Autodesk Fusion 360 part; units mm, degrees
note: some values were not read from the file. Chosen so that the rebuilt part matches the saved one: which bodies a step acts on. Set by a fixed rule: which sketch regions a step uses.
(part 6 of 6)
  spline S14 degree 5 poles (28.4182, 7.3721) (28.401, 7.3374) (28.3665, 7.2685) (28.3146, 7.1668) (28.2449, 7.0342) (28.157, 6.8738) (28.0682, 6.7185) (27.9785, 6.5686) (27.8878, 6.4239) (27.796, 6.2845) (27.7028, 6.1503) (27.6083, 6.0213) (27.5124, 5.8974) (27.4154, 5.7789) (27.3181, 5.6659) (27.2215, 5.559) (27.1271, 5.4587) (27.0359, 5.3653) (26.9485, 5.2792) (26.8646, 5.2) (26.7825, 5.127) (26.7002, 5.0594) (26.6169, 4.9965) (26.5338, 4.9388) (26.4561, 4.8881) (26.3912, 4.8473) (26.3448, 4.8184) (26.3177, 4.8012) (26.3011, 4.7914) (26.2792, 4.7817) (26.2337, 4.7638) (26.1495, 4.7307) (26.0155, 4.6776) (25.8242, 4.6008) (25.5709, 4.4983) (25.2528, 4.3688) (24.9457, 4.2431) (24.6857, 4.1365) (24.4991, 4.0599) (24.4026, 4.0202) knots 0 0 0 0 0 0 0.028571 0.057143 0.085714 0.114286 0.142857 0.171429 0.2 0.228571 0.257143 0.285714 0.314286 0.342857 0.371429 0.4 0.428571 0.457143 0.485714 0.514286 0.542857 0.571429 0.6 0.628571 0.657143 0.685714 0.714286 0.742857 0.771429 0.8 0.828571 0.857143 0.885714 0.914286 0.942857 0.971429 1 1 1 1 1 1
  arc A14 (24.4026, 4.0202) -> (27.8435, 8.3674) centre (25.5471, 6.6497) ccw
  spline S15 degree 5 poles (27.8435, 8.3674) (27.8048, 8.3699) (27.728, 8.3745) (27.6139, 8.3804) (27.4643, 8.3863) (27.2813, 8.3904) (27.1025, 8.3911) (26.9278, 8.3884) (26.7572, 8.3822) (26.5906, 8.3724) (26.4277, 8.3588) (26.2687, 8.3415) (26.1135, 8.3203) (25.9623, 8.2956) (25.8159, 8.2678) (25.675, 8.2376) (25.5409, 8.206) (25.4145, 8.1737) (25.2962, 8.1411) (25.1857, 8.108) (25.0814, 8.0734) (24.9816, 8.036) (24.8855, 7.9953) (24.794, 7.9522) (24.7113, 7.9102) (24.6435, 7.8744) (24.5952, 7.8487) (24.5668, 7.8338) (24.55, 7.8243) (24.5306, 7.8102) (24.4924, 7.7798) (24.4217, 7.7234) (24.3086, 7.6339) (24.1465, 7.5067) (23.9311, 7.3385) (23.6599, 7.1278) (23.3975, 6.9247) (23.1752, 6.7528) (23.0155, 6.6295) (22.9329, 6.5658) knots 0 0 0 0 0 0 0.028571 0.057143 0.085714 0.114286 0.142857 0.171429 0.2 0.228571 0.257143 0.285714 0.314286 0.342857 0.371429 0.4 0.428571 0.457143 0.485714 0.514286 0.542857 0.571429 0.6 0.628571 0.657143 0.685714 0.714286 0.742857 0.771429 0.8 0.828571 0.857143 0.885714 0.914286 0.942857 0.971429 1 1 1 1 1 1
  arc A15 (22.8674, 13.3435) -> (22.9329, 6.5658) centre (25.8024, 9.9826) ccw
  spline S16 degree 5 poles (22.8674, 13.3435) (22.8699, 13.3048) (22.8745, 13.228) (22.8804, 13.1139) (22.8863, 12.9643) (22.8904, 12.7813) (22.8911, 12.6025) (22.8884, 12.4278) (22.8822, 12.2572) (22.8724, 12.0906) (22.8588, 11.9277) (22.8415, 11.7687) (22.8203, 11.6135) (22.7956, 11.4623) (22.7678, 11.3159) (22.7376, 11.175) (22.706, 11.0409) (22.6737, 10.9145) (22.6411, 10.7962) (22.608, 10.6857) (22.5734, 10.5814) (22.536, 10.4816) (22.4953, 10.3855) (22.4522, 10.294) (22.4102, 10.2113) (22.3744, 10.1435) (22.3487, 10.0952) (22.3338, 10.0668) (22.3243, 10.05) (22.3102, 10.0306) (22.2798, 9.9924) (22.2234, 9.9217) (22.1339, 9.8086) (22.0067, 9.6465) (21.8385, 9.4311) (21.6278, 9.1599) (21.4247, 8.8975) (21.2528, 8.6752) (21.1295, 8.5155) (21.0658, 8.4329) knots 0 0 0 0 0 0 0.028571 0.057143 0.085714 0.114286 0.142857 0.171429 0.2 0.228571 0.257143 0.285714 0.314286 0.342857 0.371429 0.4 0.428571 0.457143 0.485714 0.514286 0.542857 0.571429 0.6 0.628571 0.657143 0.685714 0.714286 0.742857 0.771429 0.8 0.828571 0.857143 0.885714 0.914286 0.942857 0.971429 1 1 1 1 1 1
  arc A16 (21.0658, 8.4329) -> (21.8721, 13.9182) centre (20.7422, 11.2823) ccw
  spline S17 degree 5 poles (21.8721, 13.9182) (21.8374, 13.901) (21.7685, 13.8665) (21.6668, 13.8146) (21.5342, 13.7449) (21.3738, 13.657) (21.2185, 13.5682) (21.0686, 13.4785) (20.9239, 13.3878) (20.7845, 13.296) (20.6503, 13.2028) (20.5213, 13.1083) (20.3974, 13.0124) (20.2789, 12.9154) (20.1659, 12.8181) (20.059, 12.7215) (19.9587, 12.6271) (19.8653, 12.5359) (19.7792, 12.4485) (19.7, 12.3646) (19.627, 12.2825) (19.5594, 12.2002) (19.4965, 12.1169) (19.4388, 12.0338) (19.3881, 11.9561) (19.3473, 11.8912) (19.3184, 11.8448) (19.3012, 11.8177) (19.2914, 11.8011) (19.2817, 11.7792) (19.2638, 11.7337) (19.2307, 11.6495) (19.1776, 11.5155) (19.1008, 11.3242) (18.9983, 11.0709) (18.8688, 10.7528) (18.7431, 10.4457) (18.6365, 10.1857) (18.5599, 9.9991) (18.5202, 9.9026) knots 0 0 0 0 0 0 0.028571 0.057143 0.085714 0.114286 0.142857 0.171429 0.2 0.228571 0.257143 0.285714 0.314286 0.342857 0.371429 0.4 0.428571 0.457143 0.485714 0.514286 0.542857 0.571429 0.6 0.628571 0.657143 0.685714 0.714286 0.742857 0.771429 0.8 0.828571 0.857143 0.885714 0.914286 0.942857 0.971429 1 1 1 1 1 1
  arc A17 (15.0747, 15.7395) -> (18.5202, 9.9026) centre (19.2968, 14.2964) ccw
  spline S18 degree 5 poles (15.0747, 15.7395) (15.0961, 15.7073) (15.1386, 15.643) (15.2007, 15.5472) (15.2807, 15.4206) (15.3756, 15.2642) (15.4657, 15.1097) (15.5507, 14.957) (15.6306, 14.8062) (15.7054, 14.6569) (15.7751, 14.5092) (15.8396, 14.3627) (15.8989, 14.2177) (15.953, 14.0745) (16.0022, 13.9337) (16.0465, 13.7967) (16.0862, 13.6647) (16.1214, 13.5391) (16.1523, 13.4203) (16.1789, 13.3081) (16.2011, 13.2004) (16.2185, 13.0953) (16.2313, 12.9918) (16.2398, 12.891) (16.2448, 12.7983) (16.2477, 12.7217) (16.2495, 12.6671) (16.2509, 12.635) (16.2511, 12.6158) (16.2485, 12.5919) (16.2413, 12.5436) (16.2278, 12.4541) (16.2069, 12.3115) (16.1777, 12.1075) (16.1398, 11.8368) (16.0929, 11.4966) (16.0482, 11.1678) (16.0105, 10.8893) (15.9836, 10.6894) (15.9697, 10.586) knots 0 0 0 0 0 0 0.028571 0.057143 0.085714 0.114286 0.142857 0.171429 0.2 0.228571 0.257143 0.285714 0.314286 0.342857 0.371429 0.4 0.428571 0.457143 0.485714 0.514286 0.542857 0.571429 0.6 0.628571 0.657143 0.685714 0.714286 0.742857 0.771429 0.8 0.828571 0.857143 0.885714 0.914286 0.942857 0.971429 1 1 1 1 1 1
  arc A18 (15.9697, 10.586) -> (13.9253, 15.7395) centre (14.2647, 12.8919) ccw
  spline S19 degree 5 poles (13.9253, 15.7395) (13.9039, 15.7073) (13.8614, 15.643) (13.7993, 15.5472) (13.7193, 15.4206) (13.6244, 15.2642) (13.5343, 15.1097) (13.4493, 14.957) (13.3694, 14.8062) (13.2946, 14.6569) (13.2249, 14.5092) (13.1604, 14.3627) (13.1011, 14.2177) (13.047, 14.0745) (12.9978, 13.9337) (12.9535, 13.7967) (12.9138, 13.6647) (12.8786, 13.5391) (12.8477, 13.4203) (12.8211, 13.3081) (12.7989, 13.2004) (12.7815, 13.0953) (12.7687, 12.9918) (12.7602, 12.891) (12.7552, 12.7983) (12.7523, 12.7217) (12.7505, 12.6671) (12.7491, 12.635) (12.7489, 12.6158) (12.7515, 12.5919) (12.7587, 12.5436) (12.7722, 12.4541) (12.7931, 12.3115) (12.8223, 12.1075) (12.8602, 11.8368) (12.9071, 11.4966) (12.9518, 11.1678) (12.9895, 10.8893) (13.0164, 10.6894) (13.0303, 10.586) knots 0 0 0 0 0 0 0.028571 0.057143 0.085714 0.114286 0.142857 0.171429 0.2 0.228571 0.257143 0.285714 0.314286 0.342857 0.371429 0.4 0.428571 0.457143 0.485714 0.514286 0.542857 0.571429 0.6 0.628571 0.657143 0.685714 0.714286 0.742857 0.771429 0.8 0.828571 0.857143 0.885714 0.914286 0.942857 0.971429 1 1 1 1 1 1
  arc A19 (7.1279, 13.9182) -> (13.0303, 10.586) centre (11.506, 14.7795) ccw
  spline S20 degree 5 poles (7.1279, 13.9182) (7.1626, 13.901) (7.2315, 13.8665) (7.3332, 13.8146) (7.4658, 13.7449) (7.6262, 13.657) (7.7815, 13.5682) (7.9314, 13.4785) (8.0761, 13.3878) (8.2155, 13.296) (8.3497, 13.2028) (8.4787, 13.1083) (8.6026, 13.0124) (8.7211, 12.9154) (8.8341, 12.8181) (8.941, 12.7215) (9.0413, 12.6271) (9.1347, 12.5359) (9.2208, 12.4485) (9.3, 12.3646) (9.373, 12.2825) (9.4406, 12.2002) (9.5035, 12.1169) (9.5612, 12.0338) (9.6119, 11.9561) (9.6527, 11.8912) (9.6816, 11.8448) (9.6988, 11.8177) (9.7086, 11.8011) (9.7183, 11.7792) (9.7362, 11.7337) (9.7693, 11.6495) (9.8224, 11.5155) (9.8992, 11.3242) (10.0017, 11.0709) (10.1312, 10.7528) (10.2569, 10.4457) (10.3635, 10.1857) (10.4401, 9.9991) (10.4798, 9.9026) knots 0 0 0 0 0 0 0.028571 0.057143 0.085714 0.114286 0.142857 0.171429 0.2 0.228571 0.257143 0.285714 0.314286 0.342857 0.371429 0.4 0.428571 0.457143 0.485714 0.514286 0.542857 0.571429 0.6 0.628571 0.657143 0.685714 0.714286 0.742857 0.771429 0.8 0.828571 0.857143 0.885714 0.914286 0.942857 0.971429 1 1 1 1 1 1
  arc A20 (10.4798, 9.9026) -> (6.1326, 13.3435) centre (7.8503, 11.0471) ccw
  spline S21 degree 5 poles (6.1326, 13.3435) (6.1301, 13.3048) (6.1255, 13.228) (6.1196, 13.1139) (6.1137, 12.9643) (6.1096, 12.7813) (6.1089, 12.6025) (6.1116, 12.4278) (6.1178, 12.2572) (6.1276, 12.0906) (6.1412, 11.9277) (6.1585, 11.7687) (6.1797, 11.6135) (6.2044, 11.4623) (6.2322, 11.3159) (6.2624, 11.175) (6.294, 11.0409) (6.3263, 10.9145) (6.3589, 10.7962) (6.392, 10.6857) (6.4266, 10.5814) (6.464, 10.4816) (6.5047, 10.3855) (6.5478, 10.294) (6.5898, 10.2113) (6.6256, 10.1435) (6.6513, 10.0952) (6.6662, 10.0668) (6.6757, 10.05) (6.6898, 10.0306) (6.7202, 9.9924) (6.7766, 9.9217) (6.8661, 9.8086) (6.9933, 9.6465) (7.1615, 9.4311) (7.3722, 9.1599) (7.5753, 8.8975) (7.7472, 8.6752) (7.8705, 8.5155) (7.9342, 8.4329) knots 0 0 0 0 0 0 0.028571 0.057143 0.085714 0.114286 0.142857 0.171429 0.2 0.228571 0.257143 0.285714 0.314286 0.342857 0.371429 0.4 0.428571 0.457143 0.485714 0.514286 0.542857 0.571429 0.6 0.628571 0.657143 0.685714 0.714286 0.742857 0.771429 0.8 0.828571 0.857143 0.885714 0.914286 0.942857 0.971429 1 1 1 1 1 1
  arc A21 (1.1565, 8.3674) -> (7.9342, 8.4329) centre (4.5174, 11.3024) ccw
  spline S22 degree 5 poles (1.1565, 8.3674) (1.1952, 8.3699) (1.272, 8.3745) (1.3861, 8.3804) (1.5357, 8.3863) (1.7187, 8.3904) (1.8975, 8.3911) (2.0722, 8.3884) (2.2428, 8.3822) (2.4094, 8.3724) (2.5723, 8.3588) (2.7313, 8.3415) (2.8865, 8.3203) (3.0377, 8.2956) (3.1841, 8.2678) (3.325, 8.2376) (3.4591, 8.206) (3.5855, 8.1737) (3.7038, 8.1411) (3.8143, 8.108) (3.9186, 8.0734) (4.0184, 8.036) (4.1145, 7.9953) (4.206, 7.9522) (4.2887, 7.9102) (4.3565, 7.8744) (4.4048, 7.8487) (4.4332, 7.8338) (4.45, 7.8243) (4.4694, 7.8102) (4.5076, 7.7798) (4.5783, 7.7234) (4.6914, 7.6339) (4.8535, 7.5067) (5.0689, 7.3385) (5.3401, 7.1278) (5.6025, 6.9247) (5.8248, 6.7528) (5.9845, 6.6295) (6.0671, 6.5658) knots 0 0 0 0 0 0 0.028571 0.057143 0.085714 0.114286 0.142857 0.171429 0.2 0.228571 0.257143 0.285714 0.314286 0.342857 0.371429 0.4 0.428571 0.457143 0.485714 0.514286 0.542857 0.571429 0.6 0.628571 0.657143 0.685714 0.714286 0.742857 0.771429 0.8 0.828571 0.857143 0.885714 0.914286 0.942857 0.971429 1 1 1 1 1 1
  arc A22 (6.0671, 6.5658) -> (0.5818, 7.3721) centre (3.2177, 6.2422) ccw
  spline S23 degree 5 poles (0.5818, 7.3721) (0.599, 7.3374) (0.6335, 7.2685) (0.6854, 7.1668) (0.7551, 7.0342) (0.843, 6.8738) (0.9318, 6.7185) (1.0215, 6.5686) (1.1122, 6.4239) (1.204, 6.2845) (1.2972, 6.1503) (1.3917, 6.0213) (1.4876, 5.8974) (1.5846, 5.7789) (1.6819, 5.6659) (1.7785, 5.559) (1.8729, 5.4587) (1.9641, 5.3653) (2.0515, 5.2792) (2.1354, 5.2) (2.2175, 5.127) (2.2998, 5.0594) (2.3831, 4.9965) (2.4662, 4.9388) (2.5439, 4.8881) (2.6088, 4.8473) (2.6552, 4.8184) (2.6823, 4.8012) (2.6989, 4.7914) (2.7208, 4.7817) (2.7663, 4.7638) (2.8505, 4.7307) (2.9845, 4.6776) (3.1758, 4.6008) (3.4291, 4.4983) (3.7472, 4.3688) (4.0543, 4.2431) (4.3143, 4.1365) (4.5009, 4.0599) (4.5974, 4.0202) knots 0 0 0 0 0 0 0.028571 0.057143 0.085714 0.114286 0.142857 0.171429 0.2 0.228571 0.257143 0.285714 0.314286 0.342857 0.371429 0.4 0.428571 0.457143 0.485714 0.514286 0.542857 0.571429 0.6 0.628571 0.657143 0.685714 0.714286 0.742857 0.771429 0.8 0.828571 0.857143 0.885714 0.914286 0.942857 0.971429 1 1 1 1 1 1
  arc A23 (-1.2395, 0.5747) -> (4.5974, 4.0202) centre (0.2036, 4.7968) ccw
  point P0 (-0.3392, 1.1124)
  point P1 (0.4456, 1.4593)
  point P2 (1.0843, 1.6528)
  point P3 (1.5538, 1.7347)
  point P4 (1.8395, 1.7498)
  point P5 (1.9347, 1.7445)
  point P6 (-0.3392, -1.1124)
  point P7 (0.4456, -1.4593)
  point P8 (1.0843, -1.6528)
  point P9 (1.5538, -1.7347)
  point P10 (1.8395, -1.7498)
  point P11 (1.9347, -1.7445)
  point P12 (1.0927, -6.4562)
  point P13 (1.5989, -5.7634)
  point P14 (2.0552, -5.2765)
  point P15 (2.4209, -4.9708)
  point P16 (2.6607, -4.8149)
  point P17 (2.7459, -4.7719)
  point P18 (2.2051, -8.383)
  point P19 (3.0582, -8.291)
  point P20 (3.708, -8.1392)
  point P21 (4.1557, -7.9754)
  point P22 (4.4106, -7.8457)
  point P23 (4.4903, -7.7934)
  point P24 (6.117, -12.2949)
  point P25 (6.209, -11.4418)
  point P26 (6.3608, -10.792)
  point P27 (6.5246, -10.3443)
  point P28 (6.6543, -10.0894)
  point P29 (6.7066, -10.0097)
  point P30 (8.0438, -13.4073)
  point P31 (8.7366, -12.9011)
  point P32 (9.2235, -12.4448)
  point P33 (9.5292, -12.0791)
  point P34 (9.6851, -11.8393)
  point P35 (9.7281, -11.7541)
  point P36 (13.3876, -14.8392)
  point P37 (13.0407, -14.0544)
  point P38 (12.8472, -13.4157)
  point P39 (12.7653, -12.9462)
  point P40 (12.7502, -12.6605)
  point P41 (12.7555, -12.5653)
  point P42 (15.6124, -14.8392)
  point P43 (15.9593, -14.0544)
  point P44 (16.1528, -13.4157)
  point P45 (16.2347, -12.9462)
  point P46 (16.2498, -12.6605)
  point P47 (16.2445, -12.5653)
  point P48 (20.9562, -13.4073)
  point P49 (20.2634, -12.9011)
  point P50 (19.7765, -12.4448)
  point P51 (19.4708, -12.0791)
  point P52 (19.3149, -11.8393)
  point P53 (19.2719, -11.7541)
  point P54 (22.883, -12.2949)
  point P55 (22.791, -11.4418)
  point P56 (22.6392, -10.792)
  point P57 (22.4754, -10.3443)
  point P58 (22.3457, -10.0894)
  point P59 (22.2934, -10.0097)
  point P60 (26.7949, -8.383)
  point P61 (25.9418, -8.291)
  point P62 (25.292, -8.1392)
  point P63 (24.8443, -7.9754)
  point P64 (24.5894, -7.8457)
  point P65 (24.5097, -7.7934)
  point P66 (27.9073, -6.4562)
  point P67 (27.4011, -5.7634)
  point P68 (26.9448, -5.2765)
  point P69 (26.5791, -4.9708)
  point P70 (26.3393, -4.8149)
  point P71 (26.2541, -4.7719)
  point P72 (29.3392, -1.1124)
  point P73 (28.5544, -1.4593)
  point P74 (27.9157, -1.6528)
  point P75 (27.4462, -1.7347)
  point P76 (27.1605, -1.7498)
  point P77 (27.0653, -1.7445)
  point P78 (29.3392, 1.1124)
  point P79 (28.5544, 1.4593)
  point P80 (27.9157, 1.6528)
  point P81 (27.4462, 1.7347)
  point P82 (27.1605, 1.7498)
  point P83 (27.0653, 1.7445)
  point P84 (27.9073, 6.4562)
  point P85 (27.4011, 5.7634)
  point P86 (26.9448, 5.2765)
  point P87 (26.5791, 4.9708)
  point P88 (26.3393, 4.8149)
  point P89 (26.2541, 4.7719)
  point P90 (26.7949, 8.383)
  point P91 (25.9418, 8.291)
  point P92 (25.292, 8.1392)
  point P93 (24.8443, 7.9754)
  point P94 (24.5894, 7.8457)
  point P95 (24.5097, 7.7934)
  point P96 (22.883, 12.2949)
  point P97 (22.791, 11.4418)
  point P98 (22.6392, 10.792)
  point P99 (22.4754, 10.3443)
  point P100 (22.3457, 10.0894)
  point P101 (22.2934, 10.0097)
  point P102 (20.9562, 13.4073)
  point P103 (20.2634, 12.9011)
  point P104 (19.7765, 12.4448)
  point P105 (19.4708, 12.0791)
  point P106 (19.3149, 11.8393)
  point P107 (19.2719, 11.7541)
  point P108 (15.6124, 14.8392)
  point P109 (15.9593, 14.0544)
  point P110 (16.1528, 13.4157)
  point P111 (16.2347, 12.9462)
  point P112 (16.2498, 12.6605)
  point P113 (16.2445, 12.5653)
  point P114 (13.3876, 14.8392)
  point P115 (13.0407, 14.0544)
  point P116 (12.8472, 13.4157)
  point P117 (12.7653, 12.9462)
  point P118 (12.7502, 12.6605)
  point P119 (12.7555, 12.5653)
  point P120 (8.0438, 13.4073)
  point P121 (8.7366, 12.9011)
  point P122 (9.2235, 12.4448)
  point P123 (9.5292, 12.0791)
  point P124 (9.6851, 11.8393)
  point P125 (9.7281, 11.7541)
  point P126 (6.117, 12.2949)
  point P127 (6.209, 11.4418)
  point P128 (6.3608, 10.792)
  point P129 (6.5246, 10.3443)
  point P130 (6.6543, 10.0894)
  point P131 (6.7066, 10.0097)
  point P132 (2.2051, 8.383)
  point P133 (3.0582, 8.291)
  point P134 (3.708, 8.1392)
  point P135 (4.1557, 7.9754)
  point P136 (4.4106, 7.8457)
  point P137 (4.4903, 7.7934)
  point P138 (1.0927, 6.4562)
  point P139 (1.5989, 5.7634)
  point P140 (2.0552, 5.2765)
  point P141 (2.4209, 4.9708)
  point P142 (2.6607, 4.8149)
  point P143 (2.7459, 4.7719)
extrude "押し出し1''''''''''''''''" add sketch "スケッチ1 (17)" along normal blind 16 from surface at 66 separate body contours S0 A0 S1 A1 S2 A2 S3 A3 S4 A4 S5 A5 S6 A6 S7 A7 S8 A8 S9 A9 S10 A10 S11 A11 S12 A12 S13 A13 S14 A14 S15 A15 S16 A16 S17 A17 S18 A18 S19 A19 S20 A20 S21 A21 S22 A22 S23 A23 makes body 25 in component "Intermediate_Pinion_12T"
sketch "スケッチ2 (16)" plane through (0, 0, 0) normal (0, 0, 1) x (1, 0, 0) in component "Intermediate_Pinion_12T"
  circle A0 centre (14.5, 0) radius 9
extrude "押し出し2'''''''''''''''" add sketch "スケッチ2 (16)" along normal blind 4 from surface at 82 bodies 25 in component "Intermediate_Pinion_12T"
sketch "スケッチ3 (15)" plane through (0, 0, 0) normal (0, 0, 1) x (1, 0, 0) in component "Intermediate_Pinion_12T"
  circle A0 centre (14.5, 0) radius 5
extrude "押し出し3'''''''''''''" cut sketch "スケッチ3 (15)" along normal blind 30 from surface at 62 bodies 25 in component "Intermediate_Pinion_12T"
sketch "スケッチ1 (18)" plane through (0, 0, 0) normal (0, 0, 1) x (1, 0, 0) in component "Stage2_Driver_Disc"
  circle A0 centre (14.5, 0) radius 62
extrude "押し出し1'''''''''''''''''" add sketch "スケッチ1 (18)" along normal blind 14 from surface at 86 separate body makes body 26 in component "Stage2_Driver_Disc"
sketch "スケッチ2 (17)" plane through (0, 0, 0) normal (0, 0, 1) x (1, 0, 0) in component "Stage2_Driver_Disc"
  circle A0 centre (14.5, 0) radius 16
extrude "押し出し2''''''''''''''''" add sketch "スケッチ2 (17)" along normal blind 34 from surface at 86 bodies 26 in component "Stage2_Driver_Disc"
sketch "スケッチ3 (16)" plane through (0, 0, 0) normal (0, 0, 1) x (1, 0, 0) in component "Stage2_Driver_Disc"
  circle A0 centre (14.5, 0) radius 30
  circle A1 centre (-61.5, 0) radius 59
extrude "押し出し3''''''''''''''" add sketch "スケッチ3 (16)" along normal blind 20 from surface at 100 contours A0 A1 picked at (10.4448, -9.1222) bodies 26 in component "Stage2_Driver_Disc"
sketch "スケッチ4 (10)" plane through (0, 0, 0) normal (0, 0, 1) x (1, 0, 0) in component "Stage2_Driver_Disc"
  circle A0 centre (56.5, 0) radius 12
  circle A1 centre (14.5, 42) radius 12
  circle A2 centre (14.5, -42) radius 12
extrude "押し出し4''''''''" cut sketch "スケッチ4 (10)" along normal blind 14 from surface at 86 bodies 26 in component "Stage2_Driver_Disc"
sketch "スケッチ5 (8)" plane through (0, 0, 0) normal (0, 0, 1) x (1, 0, 0) in component "Stage2_Driver_Disc"
  circle A0 centre (14.5, 0) radius 5
extrude "押し出し5''''''" cut sketch "スケッチ5 (8)" along normal blind 42 from surface at 82 bodies 26 in component "Stage2_Driver_Disc"
sketch "スケッチ1 (19)" plane through (0, 0, 0) normal (0, 0, 1) x (1, 0, 0) in component "Stage2_Drive_Pin"
  circle A0 centre (-39.2401, 0) radius 6
extrude "押し出し1''''''''''''''''''" add sketch "スケッチ1 (19)" along normal blind 26 from surface at 100 separate body makes body 27 in component "Stage2_Drive_Pin"
sketch "スケッチ2 (18)" plane through (0, 0, 0) normal (0, 0, 1) x (1, 0, 0) in component "Stage2_Drive_Pin"
  circle A0 centre (-39.2401, 0) radius 9.5
extrude "押し出し2'''''''''''''''''" add sketch "スケッチ2 (18)" along normal blind 6 from surface at 120 bodies 27 in component "Stage2_Drive_Pin"
sketch "スケッチ1 (20)" plane through (0, 0, 0) normal (0, 0, 1) x (1, 0, 0) in component "Stage2_Geneva_Wheel_4Slot"
  circle A0 centre (90.5, 0) radius 58
extrude "押し出し1'''''''''''''''''''" add sketch "スケッチ1 (20)" along normal blind 12 from surface at 104 separate body makes body 28 in component "Stage2_Geneva_Wheel_4Slot"
sketch "スケッチ2 (19)" plane through (0, 0, 0) normal (0, 0, 1) x (1, 0, 0) in component "Stage2_Geneva_Wheel_4Slot"
  circle A0 centre (90.5, 0) radius 14
extrude "押し出し2''''''''''''''''''" add sketch "スケッチ2 (19)" along normal blind 18 from surface at 100 bodies 28 in component "Stage2_Geneva_Wheel_4Slot"
sketch "スケッチ3 (17)" plane through (0, 0, 0) normal (0, 0, 1) x (1, 0, 0) in component "Stage2_Geneva_Wheel_4Slot"
  line L0 (79.3561, -20.3363) -> (48.4271, -51.2652)
  line L1 (48.4271, -51.2652) -> (39.2348, -42.0729)
  line L2 (39.2348, -42.0729) -> (70.1637, -11.1439)
  arc A0 (79.3561, -20.3363) -> (70.1637, -11.1439) centre (74.7599, -15.7401) ccw
  line L3 (110.8363, -11.1439) -> (141.7652, -42.0729)
  line L4 (141.7652, -42.0729) -> (132.5729, -51.2652)
  line L5 (132.5729, -51.2652) -> (101.6439, -20.3363)
  arc A1 (110.8363, -11.1439) -> (101.6439, -20.3363) centre (106.2401, -15.7401) ccw
  line L6 (101.6439, 20.3363) -> (132.5729, 51.2652)
  line L7 (132.5729, 51.2652) -> (141.7652, 42.0729)
  line L8 (141.7652, 42.0729) -> (110.8363, 11.1439)
  arc A2 (101.6439, 20.3363) -> (110.8363, 11.1439) centre (106.2401, 15.7401) ccw
  line L9 (70.1637, 11.1439) -> (39.2348, 42.0729)
  line L10 (39.2348, 42.0729) -> (48.4271, 51.2652)
  line L11 (48.4271, 51.2652) -> (79.3561, 20.3363)
  arc A3 (70.1637, 11.1439) -> (79.3561, 20.3363) centre (74.7599, 15.7401) ccw
extrude "押し出し3'''''''''''''''" cut sketch "スケッチ3 (17)" along normal blind 20 from surface at 100 bodies 28 in component "Stage2_Geneva_Wheel_4Slot"
sketch "スケッチ4 (11)" plane through (0, 0, 0) normal (0, 0, 1) x (1, 0, 0) in component "Stage2_Geneva_Wheel_4Slot"
  circle A0 centre (166.5, 0) radius 30
  circle A1 centre (90.5, 76) radius 30
  circle A2 centre (14.5, 0) radius 30
  circle A3 centre (90.5, -76) radius 30
extrude "押し出し4'''''''''" cut sketch "スケッチ4 (11)" along normal blind 20 from surface at 100 bodies 28 in component "Stage2_Geneva_Wheel_4Slot"
sketch "スケッチ5 (9)" plane through (0, 0, 0) normal (0, 0, 1) x (1, 0, 0) in component "Stage2_Geneva_Wheel_4Slot"
  circle A0 centre (123.5, 0) radius 9
  circle A1 centre (90.5, 33) radius 9
  circle A2 centre (57.5, 0) radius 9
  circle A3 centre (90.5, -33) radius 9
extrude "押し出し5'''''''" cut sketch "スケッチ5 (9)" along normal blind 20 from surface at 100 bodies 28 in component "Stage2_Geneva_Wheel_4Slot"
sketch "スケッチ6 (4)" plane through (0, 0, 0) normal (0, 0, 1) x (1, 0, 0) in component "Stage2_Geneva_Wheel_4Slot"
  circle A0 centre (90.5, 0) radius 8
extrude "押し出し6''" cut sketch "スケッチ6 (4)" along normal blind 26 from surface at 96 bodies 28 in component "Stage2_Geneva_Wheel_4Slot"
sketch "スケッチ1 (21)" plane through (0, 0, 0) normal (0, 0, 1) x (1, 0, 0) in component "Output_Index_Table"
  circle A0 centre (90.5, 0) radius 62
extrude "押し出し1''''''''''''''''''''" add sketch "スケッチ1 (21)" along normal blind 16 from surface at 132 separate body makes body 29 in component "Output_Index_Table"
sketch "スケッチ2 (20)" plane through (0, 0, 0) normal (0, 0, 1) x (1, 0, 0) in component "Output_Index_Table"
  circle A0 centre (90.5, 0) radius 22
extrude "押し出し2'''''''''''''''''''" add sketch "スケッチ2 (20)" along normal blind 14 from surface at 118 bodies 29 in component "Output_Index_Table"
sketch "スケッチ3 (18)" plane through (0, 0, 0) normal (0, 0, 1) x (1, 0, 0) in component "Output_Index_Table"
  circle A0 centre (142.5, 0) radius 7
  circle A1 centre (132.5689, 30.5648) radius 7
  circle A2 centre (106.5689, 49.4549) radius 7
  circle A3 centre (74.4311, 49.4549) radius 7
  circle A4 centre (48.4311, 30.5648) radius 7
  circle A5 centre (38.5, 0) radius 7
  circle A6 centre (48.4311, -30.5648) radius 7
  circle A7 centre (74.4311, -49.4549) radius 7
  circle A8 centre (106.5689, -49.4549) radius 7
  circle A9 centre (132.5689, -30.5648) radius 7
extrude "押し出し3''''''''''''''''" cut sketch "スケッチ3 (18)" along normal blind 24 from surface at 128 bodies 29 in component "Output_Index_Table"
sketch "スケッチ4 (12)" plane through (0, 0, 0) normal (0, 0, 1) x (1, 0, 0) in component "Output_Index_Table"
  circle A0 centre (90.5, 0) radius 43
  circle A1 centre (90.5, 0) radius 38
extrude "押し出し4''''''''''" cut sketch "スケッチ4 (12)" along normal blind 6 from surface at 143 bodies 29 in component "Output_Index_Table"
sketch "スケッチ5 (10)" plane through (0, 0, 0) normal (0, 0, 1) x (1, 0, 0) in component "Output_Index_Table"
  circle A0 centre (116.4808, 15) radius 3.5
  circle A1 centre (90.5, 30) radius 3.5
  circle A2 centre (64.5192, 15) radius 3.5
  circle A3 centre (64.5192, -15) radius 3.5
  circle A4 centre (90.5, -30) radius 3.5
  circle A5 centre (116.4808, -15) radius 3.5
extrude "押し出し5''''''''" cut sketch "スケッチ5 (10)" along normal blind 24 from surface at 128 bodies 29 in component "Output_Index_Table"
sketch "スケッチ6 (5)" plane through (0, 0, 0) normal (0, 0, 1) x (1, 0, 0) in component "Output_Index_Table"
  circle A0 centre (90.5, 0) radius 8
extrude "押し出し6'''" cut sketch "スケッチ6 (5)" along normal blind 40 from surface at 114 bodies 29 in component "Output_Index_Table"
sketch "スケッチ1 (22)" plane through (0, 0, 0) normal (0, 0, 1) x (1, 0, 0) in component "Upper_Support_Plate"
  line L0 (-290, -125) -> (200, -125)
  line L1 (200, -125) -> (200, 125)
  line L2 (200, 125) -> (-290, 125)
  line L3 (-290, 125) -> (-290, -125)
extrude "押し出し1'''''''''''''''''''''" add sketch "スケッチ1 (22)" along normal blind 12 from surface at 158 separate body makes body 30 in component "Upper_Support_Plate"
fillet "フィレット1'" radius 24 4 edges at (-290, 125, 164) (200, 125, 164) (200, -125, 164) (-290, -125, 164) on bodies 30 in component "Upper_Support_Plate"
sketch "スケッチ2 (21)" plane through (0, 0, 0) normal (0, 0, 1) x (1, 0, 0) in component "Upper_Support_Plate"
  circle A0 centre (-176, 0) radius 12
  circle A1 centre (-80, 0) radius 11
  circle A2 centre (14.5, 0) radius 8
  circle A3 centre (90.5, 0) radius 11
extrude "押し出し2''''''''''''''''''''" cut sketch "スケッチ2 (21)" along normal blind 20 from surface at 154 bodies 30 in component "Upper_Support_Plate"
sketch "スケッチ3 (19)" plane through (0, 0, 0) normal (0, 0, 1) x (1, 0, 0) in component "Upper_Support_Plate"
  circle A0 centre (-265, 105) radius 6.5
  circle A1 centre (-265, -105) radius 6.5
  circle A2 centre (-45, 107) radius 6.5
  circle A3 centre (-45, -107) radius 6.5
  circle A4 centre (100, 107) radius 6.5
  circle A5 centre (100, -107) radius 6.5
  circle A6 centre (175, 105) radius 6.5
  circle A7 centre (175, -105) radius 6.5
extrude "押し出し3'''''''''''''''''" cut sketch "スケッチ3 (19)" along normal blind 20 from surface at 154 bodies 30 in component "Upper_Support_Plate"
sketch "スケッチ4 (13)" plane through (0, 0, 0) normal (0, 0, 1) x (1, 0, 0) in component "Upper_Support_Plate"
  circle A0 centre (-230, 0) radius 26
  circle A1 centre (150, 0) radius 26
extrude "押し出し4'''''''''''" cut sketch "スケッチ4 (13)" along normal blind 20 from surface at 154 bodies 30 in component "Upper_Support_Plate"
sketch "スケッチ1 (23)" plane through (0, 0, 0) normal (0, 0, 1) x (1, 0, 0) in component "Upper_Bearing_Rings"
  circle A0 centre (-176, 0) radius 20
  circle A1 centre (-80, 0) radius 20
  circle A2 centre (14.5, 0) radius 20
  circle A3 centre (90.5, 0) radius 20
extrude "押し出し1''''''''''''''''''''''" add sketch "スケッチ1 (23)" along normal blind 14 from surface at 170 separate body makes body 31 at (34.4006, -1.9914, 179.3333) makes body 32 at (-60.0994, -1.9914, 179.3333) makes body 33 at (-156.0994, -1.9914, 179.3333) makes body 34 at (110.4006, -1.9914, 179.3333) in component "Upper_Bearing_Rings"
sketch "スケッチ2 (22)" plane through (0, 0, 0) normal (0, 0, 1) x (1, 0, 0) in component "Upper_Bearing_Rings"
  circle A0 centre (-176, 0) radius 25
  circle A1 centre (-80, 0) radius 25
  circle A2 centre (14.5, 0) radius 25
  circle A3 centre (90.5, 0) radius 25
extrude "押し出し2'''''''''''''''''''''" add sketch "スケッチ2 (22)" along normal blind 5 from surface at 170 bodies 31 32 33 34 in component "Upper_Bearing_Rings"
sketch "スケッチ3 (20)" plane through (0, 0, 0) normal (0, 0, 1) x (1, 0, 0) in component "Upper_Bearing_Rings"
  circle A0 centre (-176, 0) radius 10.5
  circle A1 centre (-80, 0) radius 9.5
  circle A2 centre (14.5, 0) radius 6.5
  circle A3 centre (90.5, 0) radius 9.5
extrude "押し出し3''''''''''''''''''" cut sketch "スケッチ3 (20)" along normal blind 22 from surface at 166 bodies 31 32 33 34 in component "Upper_Bearing_Rings"
sketch "スケッチ1 (24)" plane through (0, 0, 0) normal (0, 0, 1) x (1, 0, 0) in component "Standoff_Bolts"
  circle A0 centre (-265, 105) radius 5.8
  circle A1 centre (-265, -105) radius 5.8
  circle A2 centre (-45, 107) radius 5.8
  circle A3 centre (-45, -107) radius 5.8
  circle A4 centre (100, 107) radius 5.8
  circle A5 centre (100, -107) radius 5.8
  circle A6 centre (175, 105) radius 5.8
  circle A7 centre (175, -105) radius 5.8
extrude "押し出し1'''''''''''''''''''''''" add sketch "スケッチ1 (24)" along normal blind 24 from surface at 146 separate body makes body 35 at (178.3857, 109.7092, 162) makes body 36 at (105.7928, 106.7109, 162) makes body 37 at (-39.2072, -107.2891, 162) makes body 38 at (-260.3766, -101.4979, 162) makes body 39 at (-39.2072, 106.7109, 162) makes body 40 at (-260.3766, 108.5021, 162) makes body 41 at (105.7928, -107.2891, 162) makes body 42 at (178.3857, -100.2908, 162) in component "Standoff_Bolts"
sketch "スケッチ2 (23)" plane through (0, 0, 0) normal (0, 0, 1) x (1, 0, 0) in component "Standoff_Bolts"
  circle A0 centre (-265, 105) radius 14
  circle A1 centre (-265, -105) radius 14
  circle A2 centre (-45, 107) radius 14
  circle A3 centre (-45, -107) radius 14
  circle A4 centre (100, 107) radius 14
  circle A5 centre (100, -107) radius 14
  circle A6 centre (175, 105) radius 14
  circle A7 centre (175, -105) radius 14
extrude "押し出し2''''''''''''''''''''''" add sketch "スケッチ2 (23)" along normal blind 3 from surface at 170 bodies 35 36 37 38 39 40 41 42 in component "Standoff_Bolts"
sketch "スケッチ3 (21)" plane through (0, 0, 0) normal (0, 0, 1) x (1, 0, 0) in component "Standoff_Bolts"
  circle A0 centre (-265, 105) radius 10.5
  circle A1 centre (-265, -105) radius 10.5
  circle A2 centre (-45, 107) radius 10.5
  circle A3 centre (-45, -107) radius 10.5
  circle A4 centre (100, 107) radius 10.5
  circle A5 centre (100, -107) radius 10.5
  circle A6 centre (175, 105) radius 10.5
  circle A7 centre (175, -105) radius 10.5
extrude "押し出し3'''''''''''''''''''" add sketch "スケッチ3 (21)" along normal blind 8 from surface at 173 bodies 35 36 37 38 39 40 41 42 in component "Standoff_Bolts"
sketch "スケッチ1 (25)" plane through (0, 0, 0) normal (0, 0, 1) x (1, 0, 0) in component "Table_Fixing_Bolts"
  circle A0 centre (116.4808, 15) radius 3.4
  circle A1 centre (90.5, 30) radius 3.4
  circle A2 centre (64.5192, 15) radius 3.4
  circle A3 centre (64.5192, -15) radius 3.4
  circle A4 centre (90.5, -30) radius 3.4
  circle A5 centre (116.4808, -15) radius 3.4
extrude "押し出し1''''''''''''''''''''''''" add sketch "スケッチ1 (25)" along normal blind 18 from surface at 130 separate body makes body 43 at (93.8958, -30.1695, 142) makes body 44 at (119.8765, 14.8305, 142) makes body 45 at (93.8958, 29.8305, 142) makes body 46 at (67.915, 14.8305, 142) makes body 47 at (66.0704, -11.9744, 142) makes body 48 at (119.8765, -15.1695, 142) in component "Table_Fixing_Bolts"
sketch "スケッチ2 (24)" plane through (0, 0, 0) normal (0, 0, 1) x (1, 0, 0) in component "Table_Fixing_Bolts"
  circle A0 centre (116.4808, 15) radius 6
  circle A1 centre (90.5, 30) radius 6
  circle A2 centre (64.5192, 15) radius 6
  circle A3 centre (64.5192, -15) radius 6
  circle A4 centre (90.5, -30) radius 6
  circle A5 centre (116.4808, -15) radius 6
extrude "押し出し2'''''''''''''''''''''''" add sketch "スケッチ2 (24)" along normal blind 5 from surface at 148 bodies 43 44 45 46 47 48 in component "Table_Fixing_Bolts"
extrude "押し出し6''''" cut sketch "スケッチ3 (14)" along normal blind 5 from surface at 66 bodies 24 in component "Intermediate_Spur_Gear_72T"
component "Lower_Base_Plate" placed x (1, 0, 0) y (0, 1, 0) z (0, 0, 1) at (0, 0, 0)
component "Bearing_Housing_A" placed x (1, 0, 0) y (0, 1, 0) z (0, 0, 1) at (0, 0, 0)
component "Bearing_Housing_B" placed x (1, 0, 0) y (0, 1, 0) z (0, 0, 1) at (0, 0, 0)
component "Bearing_Housing_C" placed x (1, 0, 0) y (0, 1, 0) z (0, 0, 1) at (0, 0, 0)
component "Bearing_Housing_D" placed x (1, 0, 0) y (0, 1, 0) z (0, 0, 1) at (0, 0, 0)
component "Standoff_Posts" placed x (1, 0, 0) y (0, 1, 0) z (0, 0, 1) at (0, 0, 0)
component "Input_Shaft" placed x (1, 0, 0) y (0, 1, 0) z (0, 0, 1) at (0, 0, 0)
component "Stage1_Shaft" placed x (1, 0, 0) y (0, 1, 0) z (0, 0, 1) at (0, 0, 0)
component "Stage2_Driver_Shaft" placed x (1, 0, 0) y (0, 1, 0) z (0, 0, 1) at (0, 0, 0)
component "Output_Shaft" placed x (1, 0, 0) y (0, 1, 0) z (0, 0, 1) at (0, 0, 0)
component "Input_Handwheel" placed x (1, 0, 0) y (0, 1, 0) z (0, 0, 1) at (0, 0, 0)
component "Input_Crank_Handle" placed x (1, 0, 0) y (0, 1, 0) z (0, 0, 1) at (0, 0, 0)
component "Stage1_Driver_Disc" placed x (1, 0, 0) y (0, 1, 0) z (0, 0, 1) at (0, 0, 0)
component "Stage1_Drive_Pin" placed x (1, 0, 0) y (0, 1, 0) z (0, 0, 1) at (0, 0, 0)
component "Stage1_Geneva_Wheel_6Slot" placed x (1, 0, 0) y (0, 1, 0) z (0, 0, 1) at (0, 0, 0)
component "Intermediate_Spur_Gear_72T" placed x (1, 0, 0) y (0, 1, 0) z (0, 0, 1) at (0, 0, 0)
component "Intermediate_Pinion_12T" placed x (1, 0, 0) y (0, 1, 0) z (0, 0, 1) at (0, 0, 0)
component "Stage2_Driver_Disc" placed x (1, 0, 0) y (0, 1, 0) z (0, 0, 1) at (0, 0, 0)
component "Stage2_Drive_Pin" placed x (1, 0, 0) y (0, 1, 0) z (0, 0, 1) at (0, 0, 0)
component "Stage2_Geneva_Wheel_4Slot" placed x (1, 0, 0) y (0, 1, 0) z (0, 0, 1) at (0, 0, 0)
component "Output_Index_Table" placed x (1, 0, 0) y (0, 1, 0) z (0, 0, 1) at (0, 0, 0)
component "Upper_Support_Plate" placed x (1, 0, 0) y (0, 1, 0) z (0, 0, 1) at (0, 0, 0)
component "Upper_Bearing_Rings" placed x (1, 0, 0) y (0, 1, 0) z (0, 0, 1) at (0, 0, 0)
component "Standoff_Bolts" placed x (1, 0, 0) y (0, 1, 0) z (0, 0, 1) at (0, 0, 0)
component "Table_Fixing_Bolts" placed x (1, 0, 0) y (0, 1, 0) z (0, 0, 1) at (0, 0, 0)
named bodies: "BasePlate", "BearingHousing_A", "BearingHousing_B", "BearingHousing_C", "BearingHousing_D", "Standoff_01", "Standoff_02", "Standoff_03", "Standoff_04", "Standoff_05", "Standoff_06", "Standoff_07", "Standoff_08", "Shaft_A", "Shaft_B", "Shaft_C", "Shaft_D", "Handwheel", "CrankHandle", "Stage1_DriverDisc", "Stage1_DrivePin", "Stage1_GenevaWheel", "Gear_72T", "Pinion_12T", "Stage2_DriverDisc", "Stage2_DrivePin", "Stage2_GenevaWheel", "Output_IndexTable", "UpperSupportPlate", "UpperBearing_A", "UpperBearing_B", "UpperBearing_C", "UpperBearing_D", "Bolt_01", "Bolt_02", "Bolt_03", "Bolt_04", "Bolt_05", "Bolt_06", "Bolt_07", "Bolt_08"
